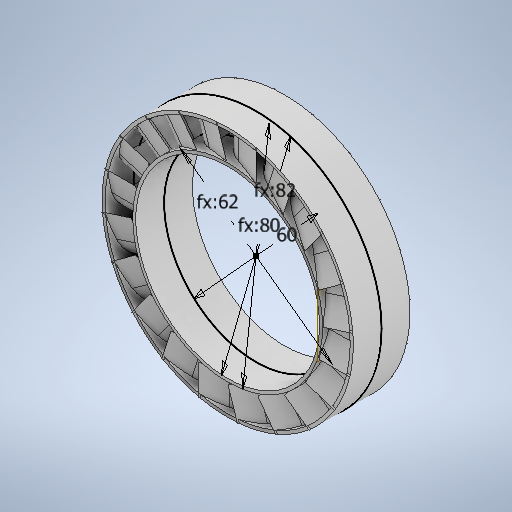
# Autodesk Inventor part: Impulse Turbine
Saved by Autodesk Inventor 2026.1 (Build 301233020, 233B)
## iProperties
Created: 2025-10-30
Part Number: Impulse Turbine
Material: Generic
Document SubType Name: Modeling
Designer: yo
Density: 1 g/cm^3
Appearance: Default
Author: yo
Autodesk Inventor part; units mm, degrees
ref_plane "XZ Plane" through (0, 0, 0) normal (0, 1, 0) x (-1, 0, 0)
ref_plane "XY Plane" through (0, 0, 0) normal (0, 0, 1) x (1, 0, 0)
ref_plane "Work Plane1" through (30, 0, 0) normal (1, 0, 0) x (0, 1, 0)
sketch "Sketch1" plane through (30, 0, 0) normal (1, 0, 0) x (0, 1, 0)
  arc A0 (4.3301, -2.5) -> (4.3301, 2.5) centre (0, 0) ccw
  arc A1 (4.3301, 2.5) -> (-1.5446, 7.1042) centre (-4.3301, -2.5) ccw
  arc A2 (-1.5446, -7.1042) -> (4.3301, -2.5) centre (-4.3301, 2.5) ccw
  line L0 (-1.5446, 7.1042) -> (-9.4819, 9.4063)
  line L1 (-1.5446, -7.1042) -> (-9.4819, -9.4063)
  arc A3 (-0.6699, 2.5) -> (-9.4819, 9.4063) centre (-13.6603, -5) ccw
  arc A4 (-0.6699, -2.5) -> (-0.6699, 2.5) centre (-5, 0) ccw
  arc A5 (-9.4819, -9.4063) -> (-0.6699, -2.5) centre (-13.6603, 5) ccw
  point P0 (0, 0)
  point P1 (5, 0)
  dimension "d1" = 5
  dimension "d2" = 10
  dimension "d4" = 5
  dimension "d6" = 5
  dimension "d7" = 10
  dimension "d8" = 5
  dimension "d9" = 15
  constraints: 14 point on circle, 7 tangent, 6 centre point, 4 end point, 2 coincident, 2 vertical alignment, 1 equal length, 1 equal radius, 1 horizontal alignment
  measures "d1" radius of A0
  measures "d2" radius of A2
  measures "d4" radius of A4
  measures "d6" distance of A1.centre A2.centre
  measures "d7" distance of A3.centre A5.centre
  measures "d8" distance of A4.centre A0.centre
  measures "d9" radius of A3
extrude "Extrusion1" add sketch "Sketch1" along normal blind 10
pattern_circular "Circular Pattern1" count 20 over 360 about axis through (0, 0, -10) along (0, 0, 1) of "Extrusion1"
sketch "Sketch2" plane through (0, 0, 0) normal (0, 0, 1) x (1, 0, 0)
  circle A0 centre (0, 0) radius 31
  circle A1 centre (0, 0) radius 30
  circle A2 centre (0, 0) radius 40
  circle A3 centre (0, 0) radius 41
  dimension "d15" = 62
  dimension "d18" = 60
  dimension "d19" = 80
  dimension "d20" = 82
  constraints: 4 centre point, 4 coincident
  measures "d15" diameter of A0
  measures "d18" diameter of A1
  measures "d19" diameter of A2
  measures "d20" diameter of A3
extrude "Extrusion2" add sketch "Sketch2" along normal mid plane 18.5
equation "\"d1\" = d6"
equation "\"d2\" = 2 * d6"
equation "\"d4\" = d6"
equation "\"d7\" = 2 * d6"
equation "\"d8\" = d6"
equation "\"d9\" = 3 * d6"
body "Solid1"
